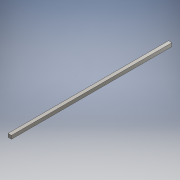
# Autodesk Inventor part: Long post for truss back
Saved by Autodesk Inventor 2016 (Build 200138000, 138)
## iProperties
Created: 2019-03-24
Part Number: Long post for truss back
Material: Stainless Steel
Document SubType Name: Modeling
Designer: benja
Density: 8 g/cm^3
Appearance: Semi-Polished
Author: benja
Autodesk Inventor part; units mm, degrees
ref_plane "YZ Plane" through (0, 0, 0) normal (1, 0, 0) x (0, 1, 0)
ref_plane "XZ Plane" through (0, 0, 0) normal (0, 1, 0) x (-1, 0, 0)
ref_plane "XY Plane" through (0, 0, 0) normal (0, 0, 1) x (1, 0, 0)
sketch "Sketch1" plane through (0, 0, 0) normal (1, 0, 0) x (0, 1, 0)
  line L0 (0, 0) -> (9440, 0)
  line L1 (9440, 0) -> (9440, -200)
  line L2 (9440, -200) -> (0, -200)
  line L3 (0, -200) -> (0, 0)
  dimension "d0" = 9440
  dimension "d1" = 200
  constraints: 8 end point, 2 parallel, 1 horizontal, 1 perpendicular
  measures "d0" distance of L1.end L2.end
  measures "d1" distance of L0.end L1.end
extrude "Extrusion1" add sketch "Sketch1" along normal blind 200
body "Solid1"
